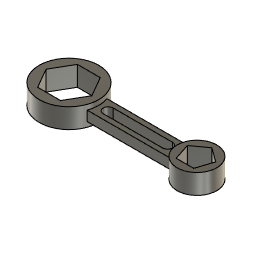
exercise 2 v2 (Autodesk Fusion 360 design; units mm, degrees)
Autodesk Fusion 360 part; units mm, degrees
sketch "Sketch1" plane through (0, 0, 0) normal (0, 0, 1) x (1, 0, 0)
  circle A0 centre (0, 0) radius 30
  line L0 (0, 0) -> (129, 0) construction
  circle A1 centre (129, 0) radius 20
  line L1 (-11.547, 20) -> (-23.094, 0)
  line L2 (-23.094, 0) -> (-11.547, -20)
  line L3 (-11.547, -20) -> (11.547, -20)
  line L4 (11.547, -20) -> (23.094, 0)
  line L5 (23.094, 0) -> (11.547, 20)
  line L6 (11.547, 20) -> (-11.547, 20)
  line L7 (0, 0) -> (0, 40) construction
  line L8 (129, 0) -> (129, 50) construction
  line L9 (129, 15) -> (114.7342, 4.6353)
  line L10 (114.7342, 4.6353) -> (120.1832, -12.1353)
  line L11 (120.1832, -12.1353) -> (137.8168, -12.1353)
  line L12 (137.8168, -12.1353) -> (143.2658, 4.6353)
  line L13 (143.2658, 4.6353) -> (129, 15)
  line L14 (28.2843, 10) -> (111.6795, 10)
  line L15 (28.2843, -10) -> (111.6795, -10)
  line L16 (30, 0) -> (109, 0) construction
  line L17 (69.5, 0) -> (69.5, 17.0528) construction
  line L18 (99.5, -5) -> (39.5, -5)
  line L19 (39.5, -5) -> (39.5, 5) construction
  line L20 (39.5, 5) -> (99.5, 5)
  line L21 (99.5, 5) -> (99.5, -5) construction
  line L22 (99.5, -5) -> (39.5, 5) construction
  line L23 (39.5, -5) -> (99.5, 5) construction
  arc A2 (39.5, 5) -> (39.5, -5) centre (39.5, 0) ccw
  arc A3 (99.5, -5) -> (99.5, 5) centre (99.5, 0) ccw
  point P0 (129, 0)
  point P1 (64.5, 0)
  point P2 (69.5, 0)
  dimension "d1" = 60
  dimension "d2" = 129
  dimension "d3" = 40
  dimension "d4" = 20
  dimension "d5" = 15
  dimension "d6" = 10
  dimension "d7" = 10
  dimension "d17" = 10
  dimension "d19" = 60
  constraint coincident A0.centre L0.start
  constraint horizontal L0
  constraint coincident P0 L0.end
  constraint perpendicular L0 L7
  constraint midpoint L6 L7
  constraint perpendicular L0 L8
  constraint coincident L8 L9.start
  constraint horizontal L14
  constraint horizontal L15
  constraint coincident A0 L16.start
  constraint coincident L0 L16.start
  constraint coincident L0 L16.end
  constraint coincident A1 L16.end
  constraint coincident L0 P2
  constraint perpendicular L14 L17
  constraint midpoint L16 P2
  constraint horizontal L18
  constraint perpendicular L18 L19
  constraint parallel L18 L20
  constraint parallel L19 L21
  constraint coincident L22 P2
  constraint coincident L23 P2
  constraint coincident P2 L17.start
  constraint coincident L16 A2.centre
  constraint tangent L20 A2
  constraint coincident L0 A3.centre
  constraint tangent L20 A3
  constraint coincident L19 A2.centre
  constraint coincident L21 A3.centre
  constraint coincident A0 L14.start
  constraint coincident A0 L15.start
  constraint coincident A1 L14.end
  constraint coincident A1 L15.end
  measures "d1" diameter of A0
  measures "d2" distance of A0.centre P0
  measures "d3" diameter of A1
  measures "d4" distance of A0.centre L6
  measures "d5" distance of L9.start P0
  measures "d6" distance of L0 L14
  measures "d7" distance of L0 L15
  measures "d17" distance of L18.end L19.end
  measures "d19" distance of L19.end L20.end
extrude "Extrude1" add sketch "Sketch1" along normal mid plane 20 contours A0 | A1 makes body 1 at (27.1662, -12.7278, 3.3333) makes body 2 at (148.9006, -1.9914, -3.3333)
extrude "Extrude2" add sketch "Sketch1" along normal mid plane 10 contours A0 A1 L14 L15 bodies 1 2
